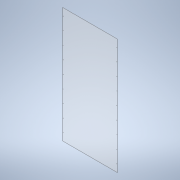
# Autodesk Inventor part: SP25V1 Acrilico
Saved by Autodesk Inventor 2021.2 (Build 252289000, 289)
## iProperties
Created: 2026-06-02
Part Number: SP25V1 Acrilico
Material: Cristal
Document SubType Name: Modeling
Designer: nelso
Density: 2.18 g/cm^3
Appearance: Transparente - Claro
Mass: 9370.9 g
Surface Area: 28808.3 cm^2
Volume: 4298.58 cm^3
Author: nelso
Autodesk Inventor part; units mm, degrees
ref_plane "YZ Plane" through (0, 0, 0) normal (1, 0, 0) x (0, 1, 0)
ref_plane "XZ Plane" through (0, 0, 0) normal (0, 1, 0) x (-1, 0, 0)
ref_plane "XY Plane" through (0, 0, 0) normal (0, 0, 1) x (1, 0, 0)
sketch "Sketch1" plane through (0, 0, 0) normal (0, 0, 1) x (1, 0, 0)
  line L0 (-390, -825) -> (390, -825)
  line L1 (390, -825) -> (390, 825)
  line L2 (390, 825) -> (-390, 825)
  line L3 (-390, 825) -> (-390, -825)
  line L4 (-390, -825) -> (390, 825) construction
  line L5 (390, -825) -> (-390, 825) construction
  point P0 (0, 0)
  dimension "d0" = 780
  dimension "d1" = 1650
  constraints: 12 end point, 2 midpoint, 2 parallel, 1 horizontal, 1 perpendicular
  measures "d0" distance of L2.end L1.end
  measures "d1" distance of L1.end L0.end
extrude "Extrusion1" add sketch "Sketch1" along normal blind 3
sketch "Sketch4" plane through (0, 0, 3) normal (0, 0, 1) x (1, 0, 0)
  line L0 (390, 825) -> (-390, 825) projected
  line L1 (0, 825) -> (-383.65, 825)
  line L2 (-383.65, 825) -> (-383.65, 720)
  point P0 (0, 0)
  point P1 (-383.65, 540)
  point P2 (-383.65, 360)
  point P3 (-383.65, 180)
  point P4 (-383.65, 0)
  point P5 (-383.65, -180)
  point P6 (-383.65, -360)
  point P7 (-383.65, -540)
  point P8 (-383.65, -720)
  point P9 (383.65, 720)
  point P10 (383.65, 540)
  point P11 (383.65, 360)
  point P12 (383.65, 180)
  point P13 (383.65, 0)
  point P14 (383.65, -180)
  point P15 (383.65, -360)
  point P16 (383.65, -540)
  point P17 (383.65, -720)
  dimension "d18" = 383.65
  dimension "d19" = 105
  dimension "d22" = 180
  dimension "d25" = 767.3
  constraints: 4 end point, 2 vertical, 1 coincident, 1 horizontal, 1 midpoint, 1 point on line, 17 other
  measures "d18" distance of L1.start L1.end
  measures "d19" distance of L1.end L2.end
  measures "d22" distance of point (-383.65, 720) point (-383.65, 540)
  measures "d25" distance of point (-383.65, 720) point (383.65, 720)
hole "Hole1" at (-383.65, 720, 3) at (-383.65, 540, 3) at (-383.65, 360, 3) at (-383.65, 180, 3) at (-383.65, 0, 3) at (-383.65, -180, 3) at (-383.65, -360, 3) at (-383.65, -540, 3) at (-383.65, -720, 3) at (383.65, 720, 3) at (383.65, 540, 3) at (383.65, 360, 3) at (383.65, 180, 3) at (383.65, 0, 3) at (383.65, -180, 3) at (383.65, -360, 3) at (383.65, -540, 3) at (383.65, -720, 3) direction (0, 0, -1) diameter 4.5 depth 8 tip angle 118 clearance for "Countersunk Flat Head Screw ISO 2009/7046" size "M4" standard "ISO"
body "Solid1"
